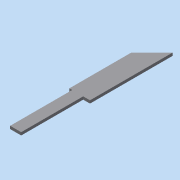
# Autodesk Inventor part: bladex1
Saved by Autodesk Inventor 2015 (Build 190159000, 159)
## iProperties
Created: 2017-09-26
Part Number: bladex1
Material: Generic
Document SubType Name: Modeling
Designer: macbook
Density: 1 g/cm^3
Appearance: Default
Author: macbook
Autodesk Inventor part; units mm, degrees
ref_plane "YZ Plane" through (0, 0, 0) normal (1, 0, 0) x (0, 1, 0)
ref_plane "XZ Plane" through (0, 0, 0) normal (0, 1, 0) x (-1, 0, 0)
ref_plane "XY Plane" through (0, 0, 0) normal (0, 0, 1) x (1, 0, 0)
sketch "Sketch1" plane through (0, 0, 0) normal (0, 0, 1) x (1, 0, 0)
  line L0 (-10, 0) -> (-10, 10)
  line L1 (0, 10) -> (0, 0)
  line L2 (-8.623, 0) -> (-8.623, -30)
  line L3 (-8.623, -30) -> (-3.288, -30)
  line L4 (-3.288, -30) -> (-3.288, 0)
  line L5 (0, 40) -> (-10, 30)
  line L6 (0, 40) -> (14.1421, 40) construction
  line L7 (-10, 30) -> (-10, 10)
  line L8 (-3.288, 0) -> (0, 0)
  line L9 (-8.623, 0) -> (-10, 0)
  line L10 (0, 40) -> (0, 10)
  dimension "d0" = 10
  dimension "d1" = 10
  dimension "d2" = 5.335
  dimension "d3" = 30
  dimension "d4" = 3.288
  dimension "d5" = 1.377
  dimension "d7" = 135
  constraints: 22 end point, 2 horizontal, 2 parallel, 2 vertical, 1 collinear, 1 equal length
  measures "d0" distance of L0.end L1.start
  measures "d1" distance of L0.start L0.end
  measures "d2" distance of L3.end L2.end
  measures "d3" distance of L2.end L2.start
  measures "d4" distance between parallel lines of L4 L1
  measures "d5" distance between parallel lines of L0 L2
  measures "d7" angle of L5 L6
extrude "Extrusion1" add sketch "Sketch1" along normal blind 1.375
body "Solid1"
